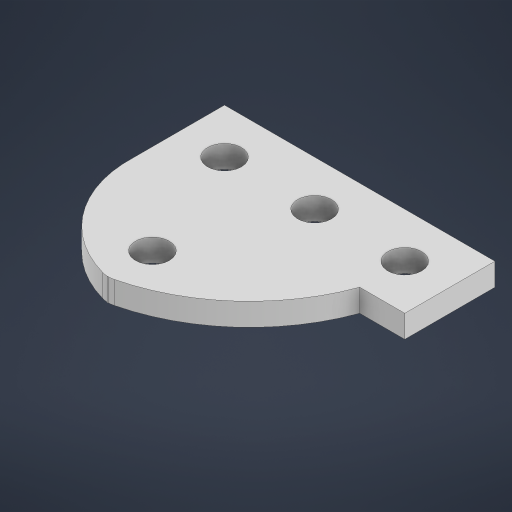
# Autodesk Inventor part: wingpiece1
Saved by Autodesk Inventor 2024 (Build 280153000, 153)
## iProperties
Created: 2023-10-22
Part Number: wingpiece1
Material: Generic
Document SubType Name: Modeling
Designer: macbook
Density: 1 g/cm^3
Appearance: Default
Author: macbook
Autodesk Inventor part; units mm, degrees
ref_plane "YZ Plane" through (0, 0, 0) normal (1, 0, 0) x (0, 1, 0)
ref_plane "XZ Plane" through (0, 0, 0) normal (0, 1, 0) x (-1, 0, 0)
ref_plane "XY Plane" through (0, 0, 0) normal (0, 0, 1) x (1, 0, 0)
sketch "Sketch1" plane through (0, 0, 0) normal (0, 1, 0) x (-1, 0, 0)
  line L0 (0, 0) -> (-38.1, 0)
  line L1 (-38.1, 0) -> (-38.1, -12.7)
  line L2 (-38.1, -12.7) -> (0, -12.7)
  line L3 (0, -12.7) -> (0, 0)
  line L4 (0, 0) -> (-12.7, 0)
  line L5 (0, 0) -> (-12.7, 0)
  line L6 (-12.7, 0) -> (-12.7, 10.16)
  line L7 (-12.7, 0) -> (-12.7, 0)
  line L8 (-12.7, 0) -> (-12.7, 10.16)
  line L9 (-12.7, 0) -> (-25.4, 0)
  line L10 (-12.7, 10.16) -> (-12.7, 16.51)
  line L11 (-12.7, 0) -> (0, -12.7)
  line L12 (-12.7, -12.7) -> (-25.4, 0)
  line L13 (-25.4, 0) -> (-25.4, -12.7)
  line L14 (-38.1, 0) -> (-25.4, -12.7)
  line L15 (-12.7, 16.51) -> (0, 0)
  line L16 (-12.7, 16.51) -> (-31.75, 0)
  arc A0 (0, 0) -> (-11.8899, 16.3095) centre (-16.1849, 0.6897) ccw
  arc A1 (-13.4792, 16.3339) -> (-31.75, 0) centre (-7.3698, -8.8856) ccw
  arc A2 (-11.8899, 16.3095) -> (-13.4792, 16.3339) centre (-12.7316, 13.2482) ccw
  point P0 (-31.75, -6.35)
  point P1 (-19.05, -6.35)
  point P2 (-6.35, -6.35)
  point P3 (-12.8011, 16.4224)
  point P4 (-12.7, 16.423)
  point P5 (-12.632, 16.4216)
  dimension "d0" = 38.1
  dimension "d1" = 12.7
  dimension "d2" = 12.7
  dimension "d3" = 12.7
  dimension "d4" = 10.16
  dimension "d6" = 12.7
  dimension "d7" = 6.35
  dimension "d20" = 3.175
  constraints: 34 end point, 8 point on circle, 6 point on line, 3 centre point, 3 midpoint, 3 parallel, 2 perpendicular, 2 tangent, 1 coincident, 1 collinear, 1 horizontal, 1 vertical
  measures "d0" distance of L2.end L1.end
  measures "d1" distance of L1.end L0.end
  measures "d2" distance of L0.start L4.end
  measures "d3" distance of L0.start L5.end
  measures "d4" distance of L5.end L6.end
  measures "d6" distance of L5.end L9.end
  measures "d7" distance of L10.start L10.end
  measures "d20" radius of A2
extrude "Extrusion1" add sketch "Sketch1" along normal blind 3.175
hole "Hole1" at (12.7, 0, 10.16) at (6.35, 0, -6.35) at (19.05, 0, -6.35) at (31.75, 0, -6.35) direction (0, 1, 0) diameter 4.7625 end through all
body "Solid1"
